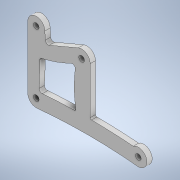
# Autodesk Inventor part: Bracket Concept MK7
Saved by Autodesk Inventor 2021 (Build 250183000, 183)
## iProperties
Created: 2021-05-11
Part Number: Bracket Concept MK7
Material: Generic
Document SubType Name: Modeling
Designer: Jawal
Density: 1 g/cm^3
Appearance: Default
Author: Jawal
Autodesk Inventor part; units mm, degrees
ref_plane "YZ Plane" through (0, 0, 0) normal (1, 0, 0) x (0, 1, 0)
ref_plane "XZ Plane" through (0, 0, 0) normal (0, 1, 0) x (-1, 0, 0)
ref_plane "XY Plane" through (0, 0, 0) normal (0, 0, 1) x (1, 0, 0)
sketch "Sketch1" plane through (0, 0, 0) normal (0, 0, 1) x (1, 0, 0)
  line L0 (-110, 70) -> (110, 70) construction
  line L1 (110, 70) -> (110, -70) construction
  line L2 (110, -70) -> (-110, -70) construction
  line L3 (-110, -70) -> (-110, 70) construction
  circle A0 centre (-90, 55) radius 5
  circle A1 centre (-90, -55) radius 5
  circle A2 centre (90, -55) radius 5
  circle A3 centre (-10, 45) radius 5
  line L4 (-67, 0) -> (-42, 0) construction
  line L5 (-42, 0) -> (-42, -30) construction
  line L6 (-42, -30) -> (-67, -30) construction
  line L7 (-67, -30) -> (-67, 0) construction
  circle A4 centre (-54.5, -11) radius 10 construction
  circle A5 centre (-63.5044, -24.4163) radius 3 construction
  circle A6 centre (-57.3559, -26.4695) radius 3 construction
  circle A7 centre (-51.263, -24.6531) radius 3 construction
  circle A8 centre (-45.3418, -26.5938) radius 3 construction
  arc A9 (-75, 54.9997) -> (-105, 55) centre (-90, 55) ccw
  arc A10 (-105, -55) -> (-90, -70) centre (-90, -55) ccw
  line L8 (-105, 55) -> (-105, -55)
  line L9 (-67.173, 37.0938) -> (-15.8457, 58.814)
  arc A11 (-80.9053, 10.3283) -> (-28.4795, 28.932) centre (-131.69, 236.6113) ccw
  arc A12 (-84.9945, -37.6763) -> (-83.834, 6.647) centre (-774.2501, 2.5469) ccw
  arc A13 (-74.1138, 41.4213) -> (-75, 54.9997) centre (-774.2501, 2.5469) ccw
  arc A14 (-74.1138, 41.4213) -> (-67.173, 37.0938) centre (-69.1215, 41.6985) ccw
  arc A15 (-80.9053, 10.3283) -> (-83.834, 6.647) centre (-80.0841, 6.6693) ccw
  arc A16 (-84.9945, -37.6763) -> (-79.3208, -42.9208) centre (-80.003, -37.9675) ccw
  arc A17 (-0.2374, 33.6118) -> (-15.8457, 58.814) centre (-10, 45) ccw
  arc A18 (87.1375, -69.7243) -> (81.0789, -42.9413) centre (90, -55) ccw
  arc A19 (90, -70) -> (-90, -70) centre (0, -989.5783) ccw
  line L10 (5, 45) -> (5, -37.2895)
  arc A20 (-21.304, 23.7513) -> (-20.2259, -37.0973) centre (169.1855, -3.3075) ccw
  line L11 (-19.6904, 33.6118) -> (-19.6904, -39.9724) construction
  line L12 (-19.6904, 33.6118) -> (53.8938, 33.6118) construction
  arc A21 (-21.304, 23.7513) -> (-28.4795, 28.932) centre (-26.2543, 24.4545) ccw
  arc A22 (-22.6296, -40.0357) -> (-20.2259, -37.0973) centre (-22.687, -37.5364) ccw
  arc A23 (5, -37.2895) -> (7.4835, -39.7895) centre (7.5, -37.2895) ccw
  arc A24 (81.0789, -42.9413) -> (7.4835, -39.7895) centre (0.7495, -1057.8516) ccw
  arc A25 (-22.6296, -40.0357) -> (-79.3208, -42.9208) centre (0.7495, -1057.8516) ccw
  point P0 (0, 0)
  point P1 (90, -70)
  dimension "d1" = 70
  dimension "d2" = 70
  dimension "d3" = 110
  dimension "d4" = 110
  dimension "d5" = 10
  dimension "d6" = 10
  dimension "d7" = 10
  dimension "d8" = 10
  dimension "d9" = 55
  dimension "d10" = 55
  dimension "d11" = 55
  dimension "d12" = 180
  dimension "d13" = 90
  dimension "d14" = 90
  dimension "d15" = 10
  dimension "d16" = 45
  dimension "d17" = 42
  dimension "d18" = 30
  dimension "d19" = 0
  dimension "d20" = 25
  dimension "d21" = 20
  dimension "d22" = 6
  dimension "d23" = 6
  dimension "d24" = 6
  dimension "d25" = 11
  dimension "d26" = 12.5
  dimension "d27" = 6
  dimension "d50" = 30
  dimension "d51" = 30
  dimension "d53" = 10
  dimension "d54" = 7.5
  dimension "d58" = 10
  dimension "d59" = 30
  dimension "d60" = 30
  dimension "d61" = 90
  dimension "d62" = 10
  dimension "d63" = 5
  dimension "d64" = 5
  constraints: 36 point on circle, 26 centre point, 26 end point, 11 tangent, 4 coincident, 4 parallel, 3 horizontal, 3 perpendicular, 2 point on line, 2 vertical
  measures "d1" distance from line of point (0, 0) L2
  measures "d2" distance from line of point (0, 0) L0
  measures "d3" distance from line of L1 point (0, 0)
  measures "d4" distance from line of point (0, 0) L3
  measures "d5" diameter of A0
  measures "d6" diameter of A1
  measures "d7" diameter of A2
  measures "d8" diameter of A3
  measures "d9" vertical distance of point (0, 0) A0.centre
  measures "d10" vertical distance of point (0, 0) A1.centre
  measures "d11" vertical distance of A2.centre point (0, 0)
  measures "d12" distance of A2.centre A1.centre
  measures "d13" horizontal distance of point (0, 0) A0.centre
  measures "d14" horizontal distance of point (0, 0) A1.centre
  measures "d15" horizontal distance of point (0, 0) A3.centre
  measures "d16" vertical distance of point (0, 0) A3.centre
  measures "d17" distance from line of point (0, 0) L5
  measures "d18" distance of L4.end L5.end
  measures "d19" distance from line of L4 point (0, 0)
  measures "d20" distance of L5.end L6.end
  measures "d21" diameter of A4
  measures "d22" diameter of A5
  measures "d23" diameter of A6
  measures "d24" diameter of A7
  measures "d25" distance from line of L4 A4.centre
  measures "d26" distance from line of L7 A4.centre
  measures "d27" diameter of A8
  measures "d50" diameter of A9
  measures "d51" diameter of A10
  measures "d53" diameter of A14
  measures "d54" diameter of A15
  measures "d58" diameter of A16
  measures "d59" diameter of A17
  measures "d60" diameter of A18
  measures "d61" angle of L11 L12
  measures "d62" diameter of A21
  measures "d63" diameter of A22
  measures "d64" diameter of A23
extrude "Extrusion5" add sketch "Sketch1" along normal blind 9.4 contours A13 A14 L9 A17 L10 A23 A24 A18 A19 A10 L8 A9
equation "\"d1\" = d2"
equation "\"d4\" = d3"
equation "\"d10\" = d9"
equation "\"d11\" = d9"
equation "\"d14\" = d13"
equation "\"d26\" = 0.5 * d20"
body "Solid5"
